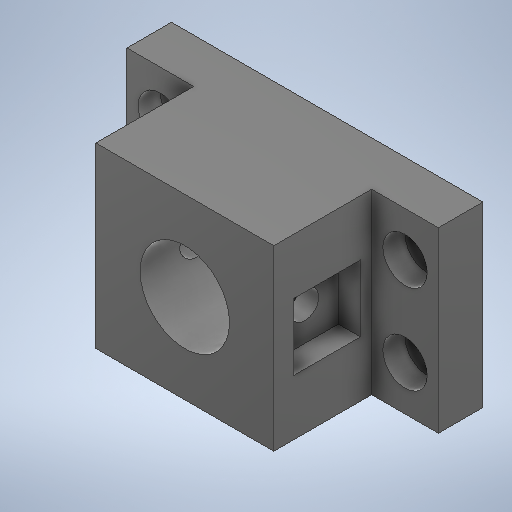
# Autodesk Inventor part: linear_bracket
Saved by Autodesk Inventor 2026.2 (Build 302298010, 298A)
## iProperties
Created: 2026-04-11
Part Number: linear_bracket
Material: ABS Plastic
Document SubType Name: Modeling
Designer: chris
Density: 1.06 g/cm^3
Appearance: Smooth - White
Author: chris
Autodesk Inventor part; units mm, degrees
ref_plane "YZ Plane" through (0, 0, 0) normal (1, 0, 0) x (0, 1, 0)
ref_plane "XZ Plane" through (0, 0, 0) normal (0, 1, 0) x (-1, 0, 0)
ref_plane "XY Plane" through (0, 0, 0) normal (0, 0, 1) x (1, 0, 0)
sketch "Sketch5" plane through (0, 0, 0) normal (0, 0, 1) x (1, 0, 0)
  line L0 (-20, -20) -> (20, -20)
  line L1 (20, -20) -> (20, 20)
  line L2 (20, 20) -> (-20, 20)
  line L3 (-20, 20) -> (-20, -20)
  line L4 (-20, -20) -> (20, 20) construction
  line L5 (20, -20) -> (-20, 20) construction
  point P0 (0, 0)
  dimension "d13" = 40
  dimension "d14" = 40
  constraints: 12 end point, 2 midpoint, 2 parallel, 1 horizontal, 1 perpendicular
  measures "d13" distance of L2.end L1.end
  measures "d14" distance of L1.end L0.end
extrude "Extrusion5" add sketch "Sketch5" against normal blind 50
sketch "Sketch6" plane through (0, 0, 0) normal (0, 0, 1) x (1, 0, 0)
  circle A0 centre (0, 0) radius 10.05
  dimension "d17" = 20.1
  constraints: 1 centre point, 1 coincident
  measures "d17" diameter of A0
extrude "Extrusion6" cut sketch "Sketch6" against normal blind 40
sketch "Sketch9" plane through (0, 0, -50) normal (0, 0, -1) x (-1, 0, 0)
  line L0 (-10.05, 10.05) -> (10.05, 10.05)
  line L1 (10.05, 10.05) -> (10.05, -10.05)
  line L2 (10.05, -10.05) -> (-10.05, -10.05)
  line L3 (-10.05, -10.05) -> (-10.05, 10.05)
  line L4 (-10.05, 10.05) -> (10.05, -10.05) construction
  line L5 (10.05, 10.05) -> (-10.05, -10.05) construction
  point P0 (0, 0)
  dimension "d28" = 20.1
  dimension "d29" = 20.1
  constraints: 12 end point, 2 midpoint, 2 parallel, 1 horizontal, 1 perpendicular
  measures "d28" distance of L1.end L2.end
  measures "d29" distance of L0.end L1.end
extrude "Extrusion9" cut sketch "Sketch9" against normal blind 5
sketch "Sketch10" plane through (20, -20, 0) normal (1, 0, 0) x (0, 0, -1)
  line L0 (40, 0) -> (50, 0)
  line L1 (50, 0) -> (50, 40)
  line L2 (50, 40) -> (40, 40)
  line L3 (40, 40) -> (40, 0)
  line L4 (40, 0) -> (50, 40) construction
  line L5 (50, 0) -> (40, 40) construction
  line L6 (50, 40) -> (50, 0) projected
  line L7 (0, 40) -> (50, 40) projected
  line L8 (0, 0) -> (50, 0) projected
  point P0 (0, 20)
  point P1 (45, 20)
  dimension "d32" = 10
  constraints: 12 end point, 3 collinear, 2 midpoint, 2 parallel, 1 horizontal, 1 perpendicular
  measures "d32" distance of L0.start L0.end
extrude "Extrusion10" add sketch "Sketch10" along normal blind 15
mirror "Mirror2" about plane through (0, 0, 0) normal (1, 0, 0) of "Extrusion10"
sketch "Sketch11" plane through (0, 0, -50) normal (0, 0, -1) x (-1, 0, 0)
  circle A0 centre (-27.5, 10) radius 2.05
  line L0 (-35, 20) -> (35, 20) projected
  line L1 (-35, -20) -> (-35, 20) projected
  circle A1 centre (-27.5, -10) radius 2.05
  circle A2 centre (27.5, -10) radius 2.05
  circle A3 centre (27.5, 10) radius 2.05
  line L2 (35, -20) -> (-35, -20) projected
  line L3 (35, -20) -> (35, 20) projected
  point P0 (0, 0)
  dimension "d35" = 4.1
  dimension "d36" = 10
  dimension "d37" = 7.5
  dimension "d38" = 4.1
  dimension "d39" = 4.1
  dimension "d41" = 4.1
  dimension "d42" = 10
  dimension "d43" = 7.5
  dimension "d44" = 7.5
  dimension "d45" = 7.5
  dimension "d46" = 10
  dimension "d47" = 10
  constraints: 4 centre point
  measures "d35" diameter of A0
  measures "d36" distance from line of L0 A0.centre
  measures "d37" distance from line of L1 A0.centre
  measures "d38" diameter of A1
  measures "d39" diameter of A2
  measures "d41" diameter of A3
  measures "d42" distance from line of L2 A1.centre
  measures "d43" distance from line of L1 A1.centre
  measures "d44" distance from line of L3 A3.centre
  measures "d45" distance from line of L3 A2.centre
  measures "d46" distance from line of L2 A2.centre
  measures "d47" distance from line of L0 A3.centre
extrude "Extrusion11" cut sketch "Sketch11" against normal through all contours A0 | A1 | A2 | A3
sketch "Sketch12" plane through (20, -20, -40) normal (0, 0, 1) x (1, 0, 0)
  circle A0 centre (7.5, 30) radius 2.05 projected
  circle A1 centre (7.5, 10) radius 2.05 projected
  circle A2 centre (-47.5, 10) radius 2.05 projected
  circle A3 centre (-47.5, 30) radius 2.05 projected
  circle A4 centre (7.5, 30) radius 5
  circle A5 centre (7.5, 10) radius 5
  circle A6 centre (-47.5, 30) radius 5
  circle A7 centre (-47.5, 10) radius 5
  point P0 (-20, 20)
  dimension "d50" = 10
  dimension "d51" = 10
  dimension "d52" = 10
  dimension "d53" = 10
  constraints: 4 centre point, 4 coincident
  measures "d50" diameter of A4
  measures "d51" diameter of A5
  measures "d52" diameter of A6
  measures "d53" diameter of A7
extrude "Extrusion12" cut sketch "Sketch12" against normal blind 5
sketch "Sketch13" plane through (20, -20, 0) normal (1, 0, 0) x (0, 0, -1)
  circle A0 centre (30, 20) radius 3.1
  line L0 (40, 40) -> (40, 0) projected
  point P0 (0, 20)
  point P1 (40, 20)
  dimension "d56" = 6.2
  dimension "d57" = 10
  constraints: 1 centre point, 1 midpoint
  measures "d56" diameter of A0
  measures "d57" distance of point (40, 20) A0.centre
extrude "Extrusion13" cut sketch "Sketch13" against normal through all
sketch "Sketch14" plane through (20, -20, 0) normal (1, 0, 0) x (0, 0, -1)
  line L0 (37.5, 27.5) -> (22.5, 27.5)
  line L1 (22.5, 27.5) -> (22.5, 12.5)
  line L2 (22.5, 12.5) -> (37.5, 12.5)
  line L3 (37.5, 12.5) -> (37.5, 27.5)
  line L4 (37.5, 27.5) -> (22.5, 12.5) construction
  line L5 (22.5, 27.5) -> (37.5, 12.5) construction
  line L6 (40, 0) -> (40, 40) projected
  circle A0 centre (30, 20) radius 3.1 projected
  point P0 (0, 20)
  dimension "d60" = 15
  dimension "d61" = 15
  constraints: 12 end point, 2 midpoint, 2 parallel, 1 coincident, 1 horizontal, 1 perpendicular
  measures "d60" distance of L2.end L1.end
  measures "d61" distance of L1.end L0.end
extrude "Extrusion14" cut sketch "Sketch14" against normal blind 5 contours L3 L2 L1 L0 | A0
mirror "Mirror3" about plane through (0, 0, 0) normal (1, 0, 0) of "Extrusion14"
sketch "Sketch15" plane through (0, 0, 0) normal (0, 0, 1) x (1, 0, 0)
  line L0 (-20, -20) -> (20, -20)
  line L1 (20, -20) -> (20, 20)
  line L2 (20, 20) -> (-20, 20)
  line L3 (-20, 20) -> (-20, -20)
  line L4 (-20, -20) -> (20, 20) construction
  line L5 (20, -20) -> (-20, 20) construction
  circle A0 centre (0, 0) radius 10.05 projected
  circle A1 centre (0, 0) radius 10.05
  line L6 (20, 20) -> (-20, 20) projected
  line L7 (-20, 20) -> (-20, -20) projected
  line L8 (-20, -20) -> (20, -20) projected
  line L9 (20, -20) -> (20, 20) projected
  constraints: 12 end point, 4 collinear, 2 parallel, 1 centre point, 1 coincident, 1 concentric, 1 horizontal, 1 perpendicular
extrude "Extrusion15" cut sketch "Sketch15" against normal blind 18
body "Solid2"
